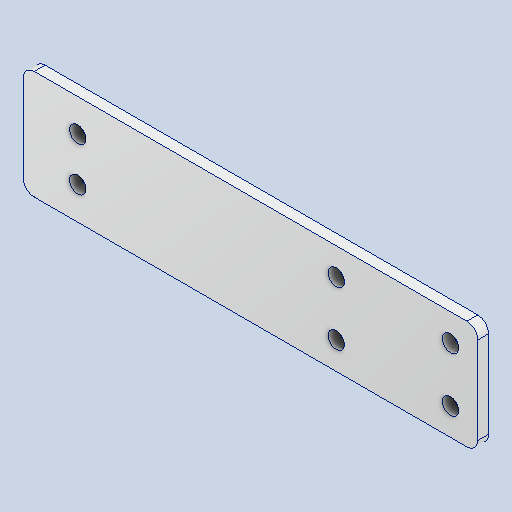
# Autodesk Inventor part: dribl-v4-Plate-4
Saved by Autodesk Inventor 2025.2 (Build 292293000, 293)
## iProperties
Created: 2025-05-15
Part Number: dribl-v4-Plate-4
Material: アルミニウム 6061
Document SubType Name: Modeling
Designer: haruy
Density: 2.7 g/cm^3
Appearance: アルミニウム - フラット
Author: haruy
Autodesk Inventor part; units mm, degrees
ref_plane "YZ Plane" through (0, 0, 0) normal (1, 0, 0) x (0, 1, 0)
ref_plane "XZ Plane" through (0, 0, 0) normal (0, 1, 0) x (-1, 0, 0)
ref_plane "XY Plane" through (0, 0, 0) normal (0, 0, 1) x (1, 0, 0)
derived "dribl-v3-Sketch-Base.ipt"
sketch "スケッチ15" plane through (400, -432.3334, -303) normal (0, 0, 1) x (1, 0, 0)
  line L0 (-20, 0) -> (-20, 1437.5) projected
  line L1 (-20, 1412.5) -> (0, 1412.5) projected
  line L2 (0, 1437.5) -> (0, 0) projected
  line L3 (0, 1437.5) -> (-20, 1437.5) projected
  circle A0 centre (-10, 1374.5) radius 1.5 projected
  circle A1 centre (-10, 1366.5) radius 1.5 projected
  line L4 (-20, 516.5) -> (0, 516.5) projected
  line L5 (0, 0) -> (-20, 0) projected
  circle A2 centre (-10, 503.5) radius 1.5 projected
  circle A3 centre (-10, 495.5) radius 1.5 projected
  line L6 (-580, 268) -> (-20, 268) projected
  line L7 (-300, 268) -> (-300, 248) projected
  line L8 (-580, 248) -> (-20, 248) projected
  circle A4 centre (-590, 503.5) radius 1.5 projected
  circle A5 centre (-590, 495.5) radius 1.5 projected
  circle A6 centre (-590, 1366.5) radius 1.5 projected
  circle A7 centre (-590, 1374.5) radius 1.5 projected
  line L9 (-600, 1437.5) -> (-600, 0) projected
  line L10 (-600, 438) -> (-580, 438) projected
  line L11 (-600, 348) -> (-580, 348) projected
  line L12 (-600, 428) -> (-433.1583, 428) projected
  line L13 (-547.5, 428) -> (-516.5, 428) projected
  line L14 (-516.5, 428) -> (-516.5, 408) projected
  line L15 (-516.5, 408) -> (-547.5, 408) projected
  line L16 (-547.5, 408) -> (-547.5, 428) projected
  circle A8 centre (-542.5, 423) radius 1.5 projected
  circle A9 centre (-521.5, 423) radius 1.5 projected
  circle A10 centre (-542.5, 413) radius 1.5 projected
  circle A11 centre (-521.5, 413) radius 1.5 projected
  line L17 (-532, 428) -> (-532, 408) projected
  line L18 (-580, 0) -> (-580, 1437.5) projected
  line L19 (-547.5, 408) -> (-600, 408) projected
  line L20 (-600, 428) -> (-600, 408) projected
  circle A12 centre (-590, 422) radius 1.5 projected
  circle A13 centre (-590, 414) radius 1.5 projected
  point P0 (-400, 432.3334)
extrude "押し出し1" add sketch "スケッチ15" against normal blind 2 contours L12 L18 L19 L9 | L12 L16 L19 L18 | L12 L17 L15 L16 | L12 L14 L15 L17
fillet "フィレット1" radius 2 4 edges at (-200, -4.3334, -304) (-200, -24.3334, -304) (-116.5, -24.3334, -304) (-116.5, -4.3334, -304)
